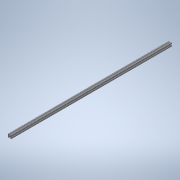
# Autodesk Inventor part: 1003-48-CL
Saved by Autodesk Inventor 2020 (Build 240168000, 168)
## iProperties
Created: 2020-01-07
Part Number: 1003-48-CL
Material: Generic
Catalog Web Link: www.cadenas.de
Description: 1003, 1003-Black-FB-T-Slotted Profile - 10 Series
Vendor: 8020
Document SubType Name: Modeling
Designer: psadmin
Manufacturer: 8020
Mass: 360.964 g
Surface Area: 2860.21 cm^2
Volume: 360.964 cm^3
Density: 1 g/cm^3
Appearance: PSOLRGB-191-191-191
Category: PARTsolutions
Company: 8020
PSOL_IDENT_0: {$CADENAS_DATA\23d-libs\8020\inch\profiles\10_series\1003.prj},182 {VTYP=3D},{NB=1003-48-CL},{LINA=1
PSOL_IDENT_1: 003-48},{NN=1003, 1003-Black-FB},{DATE=01.10.2019 06:04:27},{GEOMDATE=09.02.2018 14:25:06},{VERSION=
PSOL_IDENT_2: },{LINEID=10},{WBVAR=FINISH,LS,L},{WBNUMERIC=L}  {NB=1003-48-CL},{LINA=1003-48},{KT=DUMMY},{PN=1003-
PSOL_IDENT_3: 48},{SERIES=1003},{MAT=6105-T5 Aluminum},{FINISH=CA},{LS=-CL},{L=48.000},{LALG=[1:242/0.005]},{W=.53
PSOL_IDENT_4: 33},{MIX=.0441},{MIY=.0491},{EA=.4582},{CLR=.75,.75,.75}
NN: 1003, 1003-Black-FB
NT: T-Slotted Profile - 10 Series
NB: 1003-48-CL
NBSYN: $PN.$LS.
LINA: 1003-48
PN: 1003-48
SERIES: 1003
MAT: 6105-T5 Aluminum
FINISH: Clear Anodize
LS: Custom Length
L: 48
W: .5333
MIX: .0441
MIY: .0491
EA: .4582
SUPPLIER: 8020
ARTICLENO: 1003-48-CL
BOMINFO: 1003-48
CREATOR: CADENAS GmbH
Title: 1003-48
Author: Cadenas PARTsolutions
Comments: T-Slotted Profile - 10 Series
Autodesk Inventor part; units mm, degrees
ref_plane "YZ Plane" through (0, 0, 0) normal (1, 0, 0) x (0, 1, 0)
ref_plane "XZ Plane" through (0, 0, 0) normal (0, 1, 0) x (-1, 0, 0)
ref_plane "XY Plane" through (0, 0, 0) normal (0, 0, 1) x (1, 0, 0)
sketch "Sketch_1" plane through (0, 0, 0) normal (0, 0, 1) x (1, 0, 0)
  arc A0 (-12.7, -10.5664) -> (-10.5664, -12.7) centre (-10.592, -10.592) ccw
  arc A1 (-9.5504, -12.7) -> (-10.5664, -12.7) centre (-10.0584, -12.7) ccw
  line L0 (-9.5504, -12.7) -> (-6.3246, -12.7)
  arc A2 (-5.3086, -12.7) -> (-6.3246, -12.7) centre (-5.8166, -12.7) ccw
  line L1 (-5.3086, -12.7) -> (-4.3023, -12.7)
  arc A3 (-4.3023, -12.7) -> (-4.3023, -10.4902) centre (-4.3023, -11.5951) ccw
  line L2 (-4.3023, -10.4902) -> (-6.4748, -10.4902)
  arc A4 (-7.1932, -8.7558) -> (-6.4748, -10.4902) centre (-6.4748, -9.4742) ccw
  line L3 (-7.1932, -8.7558) -> (-3.8759, -5.4384)
  arc A5 (-1.6308, -4.5085) -> (-3.8759, -5.4384) centre (-1.6308, -7.6835) ccw
  line L4 (-1.6308, -4.5085) -> (1.6308, -4.5085)
  arc A6 (3.8759, -5.4384) -> (1.6308, -4.5085) centre (1.6308, -7.6835) ccw
  line L5 (3.8759, -5.4384) -> (7.1932, -8.7558)
  arc A7 (6.4748, -10.4902) -> (7.1932, -8.7558) centre (6.4748, -9.4742) ccw
  line L6 (6.4748, -10.4902) -> (4.3023, -10.4902)
  arc A8 (4.3023, -10.4902) -> (4.3023, -12.7) centre (4.3023, -11.5951) ccw
  line L7 (4.3023, -12.7) -> (5.3086, -12.7)
  arc A9 (6.3246, -12.7) -> (5.3086, -12.7) centre (5.8166, -12.7) ccw
  line L8 (6.3246, -12.7) -> (9.5504, -12.7)
  arc A10 (10.5664, -12.7) -> (9.5504, -12.7) centre (10.0584, -12.7) ccw
  arc A11 (10.5664, -12.7) -> (12.7, -10.5664) centre (10.592, -10.592) ccw
  arc A12 (12.7, -9.5504) -> (12.7, -10.5664) centre (12.7, -10.0584) ccw
  line L9 (12.7, -9.5504) -> (12.7, -6.3246)
  arc A13 (12.7, -5.3086) -> (12.7, -6.3246) centre (12.7, -5.8166) ccw
  line L10 (12.7, -5.3086) -> (12.7, -4.3023)
  arc A14 (12.7, -4.3023) -> (10.4902, -4.3023) centre (11.5951, -4.3023) ccw
  line L11 (10.4902, -4.3023) -> (10.4902, -6.4748)
  arc A15 (8.7558, -7.1932) -> (10.4902, -6.4748) centre (9.4742, -6.4748) ccw
  line L12 (8.7558, -7.1932) -> (5.4384, -3.8759)
  arc A16 (4.5085, -1.6308) -> (5.4384, -3.8759) centre (7.6835, -1.6308) ccw
  line L13 (4.5085, -1.6308) -> (4.5085, 1.6308)
  arc A17 (5.4384, 3.8759) -> (4.5085, 1.6308) centre (7.6835, 1.6308) ccw
  line L14 (5.4384, 3.8759) -> (8.7558, 7.1932)
  arc A18 (10.4902, 6.4748) -> (8.7558, 7.1932) centre (9.4742, 6.4748) ccw
  line L15 (10.4902, 6.4748) -> (10.4902, 4.3023)
  arc A19 (10.4902, 4.3023) -> (12.7, 4.3023) centre (11.5951, 4.3023) ccw
  line L16 (12.7, 4.3023) -> (12.7, 5.3086)
  arc A20 (12.7, 6.3246) -> (12.7, 5.3086) centre (12.7, 5.8166) ccw
  line L17 (12.7, 6.3246) -> (12.7, 9.5504)
  arc A21 (12.7, 10.5664) -> (12.7, 9.5504) centre (12.7, 10.0584) ccw
  arc A22 (12.7, 10.5664) -> (10.5664, 12.7) centre (10.592, 10.592) ccw
  arc A23 (9.5504, 12.7) -> (10.5664, 12.7) centre (10.0584, 12.7) ccw
  line L18 (9.5504, 12.7) -> (6.3246, 12.7)
  arc A24 (5.3086, 12.7) -> (6.3246, 12.7) centre (5.8166, 12.7) ccw
  line L19 (5.3086, 12.7) -> (4.3023, 12.7)
  arc A25 (4.3023, 12.7) -> (4.3023, 10.4902) centre (4.3023, 11.5951) ccw
  line L20 (4.3023, 10.4902) -> (6.4748, 10.4902)
  arc A26 (7.1932, 8.7558) -> (6.4748, 10.4902) centre (6.4748, 9.4742) ccw
  line L21 (7.1932, 8.7558) -> (3.8759, 5.4384)
  arc A27 (1.6308, 4.5085) -> (3.8759, 5.4384) centre (1.6308, 7.6835) ccw
  line L22 (1.6308, 4.5085) -> (-1.6308, 4.5085)
  arc A28 (-3.8759, 5.4384) -> (-1.6308, 4.5085) centre (-1.6308, 7.6835) ccw
  line L23 (-3.8759, 5.4384) -> (-7.1932, 8.7558)
  arc A29 (-6.4748, 10.4902) -> (-7.1932, 8.7558) centre (-6.4748, 9.4742) ccw
  line L24 (-6.4748, 10.4902) -> (-4.3023, 10.4902)
  arc A30 (-4.3023, 10.4902) -> (-4.3023, 12.7) centre (-4.3023, 11.5951) ccw
  line L25 (-4.3023, 12.7) -> (-5.3086, 12.7)
  arc A31 (-6.3246, 12.7) -> (-5.3086, 12.7) centre (-5.8166, 12.7) ccw
  line L26 (-6.3246, 12.7) -> (-9.5504, 12.7)
  arc A32 (-10.5664, 12.7) -> (-9.5504, 12.7) centre (-10.0584, 12.7) ccw
  arc A33 (-10.5664, 12.7) -> (-12.7, 10.5664) centre (-10.592, 10.592) ccw
  arc A34 (-12.7, 9.5504) -> (-12.7, 10.5664) centre (-12.7, 10.0584) ccw
  line L27 (-12.7, 9.5504) -> (-12.7, 6.3246)
  arc A35 (-12.7, 5.3086) -> (-12.7, 6.3246) centre (-12.7, 5.8166) ccw
  line L28 (-12.7, 5.3086) -> (-12.7, -5.3086)
  arc A36 (-12.7, -6.3246) -> (-12.7, -5.3086) centre (-12.7, -5.8166) ccw
  line L29 (-12.7, -6.3246) -> (-12.7, -9.5504)
  arc A37 (-12.7, -10.5664) -> (-12.7, -9.5504) centre (-12.7, -10.0584) ccw
  circle A38 centre (0, 0) radius 2.6035
  arc A39 (-10.4902, -6.4135) -> (-9.4742, -7.4295) centre (-9.4742, -6.4135) ccw
  arc A40 (-9.4742, -7.4295) -> (-8.6945, -7.1319) centre (-9.4638, -6.2865) ccw
  line L30 (-8.6945, -7.1319) -> (-5.4384, -3.8759)
  arc A41 (-5.4384, -3.8759) -> (-4.5085, -1.6308) centre (-7.6835, -1.6308) ccw
  line L31 (-4.5085, -1.6308) -> (-4.5085, 1.6308)
  arc A42 (-4.5085, 1.6308) -> (-5.4384, 3.8759) centre (-7.6835, 1.6308) ccw
  line L32 (-5.4384, 3.8759) -> (-8.6945, 7.1319)
  arc A43 (-8.6945, 7.1319) -> (-9.4742, 7.4295) centre (-9.4638, 6.2865) ccw
  arc A44 (-9.4742, 7.4295) -> (-10.4902, 6.4135) centre (-9.4742, 6.4135) ccw
  line L33 (-10.4902, 6.4135) -> (-10.4902, -6.4135)
  constraints: 88 point on circle, 68 end point, 45 centre point
extrude "Extrusion1" add sketch "Sketch_1" against normal blind 1219.2
body "Solid1"
